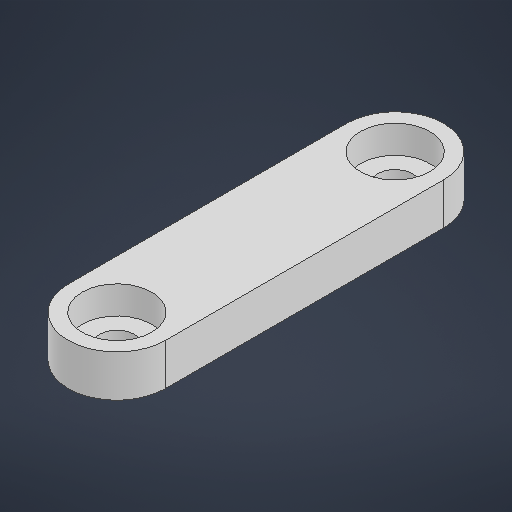
# Autodesk Inventor part: Link
Saved by Autodesk Inventor 2025.1 (Build 291241000, 241)
## iProperties
Created: 2025-03-13
Part Number: Link
Material: Generic
Document SubType Name: Modeling
Designer: jerem
Density: 1 g/cm^3
Appearance: Default
Author: jerem
## iProperties of the stored document Link_3DPrint.ipt
Created: 2025-03-13
Part Number: Link_3DPrint
Material: Generic
Document SubType Name: Modeling
Designer: jerem
Density: 1 g/cm^3
Appearance: Default
Author: jerem
Autodesk Inventor part; units mm, degrees
ref_plane "YZ Plane" through (0, 0, 0) normal (1, 0, 0) x (0, 1, 0)
ref_plane "XZ Plane" through (0, 0, 0) normal (0, 1, 0) x (-1, 0, 0)
ref_plane "XY Plane" through (0, 0, 0) normal (0, 0, 1) x (1, 0, 0)
sketch "Sketch1" plane through (0, 0, 0) normal (0, 1, 0) x (-1, 0, 0)
  circle A0 centre (0, 0) radius 3.5
  circle A1 centre (0, -20) radius 3.5
  line L0 (3.5, 0) -> (3.5, -20)
  line L1 (-3.5, -20) -> (-3.5, 0)
  line L2 (0, 0) -> (0, -20) construction
  circle A2 centre (0, 0) radius 1.25
  circle A3 centre (0, -20) radius 1.25
  circle A4 centre (0, -20) radius 2.5
  circle A5 centre (0, 0) radius 2.5
  dimension "d0" = 7
  dimension "d1" = 2.5
  dimension "d2" = 20
  dimension "d5" = 5
  dimension "d6" = 5
  constraints: 6 centre point, 6 end point, 5 coincident, 4 point on circle, 4 tangent, 2 equal radius, 1 vertical
  measures "d0" diameter of A0
  measures "d1" diameter of A2
  measures "d2" distance of L2.start L2.end
  measures "d5" diameter of A4
  measures "d6" diameter of A5
extrude "Extrusion1" add sketch "Sketch1" along normal blind 3 contours A0 | L0 A1 L1 A0 | A1
extrude "Extrusion2" add sketch "Sketch1" along normal blind 1 contours A4 | A5
body "Solid1"
